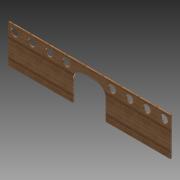
# Autodesk Inventor part: manipulator back pannel 2
Saved by Autodesk Inventor 2012 (Build 160160000, 160)
## iProperties
Created: 2013-09-02
Part Number: manipulator back pannel 2
Material: Default
Document SubType Name: Modeling
Designer: Bryce
Density: 1 g/cm^3
Author: Bryce
Autodesk Inventor part; units mm, degrees
ref_plane "YZ Plane" through (0, 0, 0) normal (1, 0, 0) x (0, 1, 0)
ref_plane "XZ Plane" through (0, 0, 0) normal (0, 1, 0) x (-1, 0, 0)
ref_plane "XY Plane" through (0, 0, 0) normal (0, 0, 1) x (1, 0, 0)
sketch "Sketch1" plane through (0, 0, 0) normal (0, 0, 1) x (1, 0, 0)
  line L0 (812.8, 0) -> (812.8, 190.5)
  line L1 (812.8, 190.5) -> (0, 190.5)
  line L2 (0, 190.5) -> (0, 0)
  circle A0 centre (781.05, 158.75) radius 19.05
  circle A1 centre (520.7, 158.75) radius 19.05
  circle A2 centre (292.1, 158.75) radius 19.05
  circle A3 centre (31.75, 158.75) radius 19.05
  circle A4 centre (694.2667, 158.75) radius 19.05
  circle A5 centre (205.3167, 158.75) radius 19.05
  circle A6 centre (607.4833, 158.75) radius 19.05
  circle A7 centre (118.5333, 158.75) radius 19.05
  line L3 (488.95, 0) -> (488.95, 101.6)
  line L4 (488.95, 152.4) -> (438.15, 152.4) construction
  line L5 (323.85, 152.4) -> (323.85, 101.6) construction
  line L6 (0, 0) -> (323.85, 0)
  line L7 (488.95, 0) -> (812.8, 0)
  arc A8 (374.65, 152.4) -> (323.85, 101.6) centre (374.65, 101.6) ccw
  arc A9 (488.95, 101.6) -> (438.15, 152.4) centre (438.15, 101.6) ccw
  line L8 (374.65, 152.4) -> (323.85, 152.4) construction
  line L9 (323.85, 101.6) -> (323.85, 0)
  line L10 (438.15, 152.4) -> (374.65, 152.4)
  line L11 (488.95, 101.6) -> (488.95, 152.4) construction
  dimension "d0" = 190.5
  dimension "d1" = 812.8
  dimension "d13" = 38.1
  dimension "d14" = 38.1
  dimension "d15" = 228.6
  dimension "d16" = 260.35
  dimension "d17" = 86.7833
  dimension "d18" = 86.7833
  dimension "d21" = 31.75
  dimension "d22" = 31.75
  dimension "d23" = 31.75
  dimension "d24" = 86.7833
  dimension "d25" = 86.7833
  dimension "d26" = 165.1
  dimension "d28" = 323.85
  dimension "d29" = 152.4
  dimension "d30" = 50.8
  constraints: 24 end point, 10 centre point, 10 tangent, 8 perpendicular, 7 equal radius, 7 horizontal alignment, 7 parallel, 4 point on circle, 2 horizontal, 1 coincident, 1 collinear
  measures "d0" distance of L1.end L2.end
  measures "d1" distance of L0.end L1.end
  measures "d13" diameter of A0
  measures "d14" diameter of A1
  measures "d15" distance of A2.centre A1.centre
  measures "d16" distance of A1.centre A0.centre
  measures "d17" distance of A4.centre A0.centre
  measures "d18" distance of A5.centre A2.centre
  measures "d21" distance from line of L1 A3.centre
  measures "d22" distance from line of L2 A3.centre
  measures "d23" distance from line of L0 A0.centre
  measures "d24" distance of A6.centre A4.centre
  measures "d25" distance of A7.centre A5.centre
  measures "d26" distance of L4.start L5.start
  measures "d28" distance between parallel lines of L2 L5
  measures "d29" distance of L5.start L6.end
  measures "d30" radius of A8
extrude "Extrusion1" add sketch "Sketch1" along normal blind 6.35
equation "\"d14\" = d13"
equation "\"d16\" = 0.5 * d1 - 0.5 * d15 - d23"
equation "\"d17\" = 0.333333 * d16"
equation "\"d18\" = d17"
equation "\"d23\" = d22"
equation "\"d24\" = d17"
equation "\"d25\" = d18"
equation "\"d28\" = -0.5 * d26 + 0.5 * d1"
body "Solid1"
